Autodesk Fusion 360 part; units mm, degrees
(part 3 of 3)
  spline S38 degree 5 poles (8.1024, -6.5353) (8.1055, -6.5377) (8.1117, -6.5426) (8.1212, -6.5498) (8.1342, -6.5589) (8.1508, -6.5697) (8.1678, -6.5801) (8.1849, -6.5902) (8.2022, -6.6002) (8.2195, -6.6101) (8.237, -6.6198) (8.2545, -6.6295) (8.2721, -6.639) (8.2899, -6.6483) (8.3078, -6.6574) (8.3259, -6.6663) (8.3441, -6.6751) (8.3624, -6.6837) (8.3807, -6.6922) (8.3992, -6.7006) (8.4177, -6.7089) (8.4363, -6.717) (8.455, -6.725) (8.4738, -6.7329) (8.4927, -6.7407) (8.5116, -6.7484) (8.5307, -6.7559) (8.5498, -6.7633) (8.569, -6.7706) (8.5882, -6.7778) (8.6075, -6.7849) (8.6269, -6.7919) (8.6464, -6.7988) (8.6659, -6.8056) (8.6855, -6.8123) (8.7052, -6.8189) (8.7249, -6.8254) (8.7447, -6.8318) (8.7645, -6.838) (8.7845, -6.8442) (8.8044, -6.8503) (8.8245, -6.8563) (8.8446, -6.8622) (8.8647, -6.868) (8.8849, -6.8737) (8.9052, -6.8794) (8.9255, -6.8849) (8.9459, -6.8903) (8.9663, -6.8957) (8.9868, -6.9009) (9.0073, -6.9061) (9.0279, -6.9112) (9.0485, -6.9162) (9.0692, -6.9211) (9.0899, -6.9259) (9.1107, -6.9306) (9.1316, -6.9352) (9.1524, -6.9398) (9.1734, -6.9442) (9.1944, -6.9486) (9.2154, -6.9529) (9.2365, -6.9571) (9.2576, -6.9613) (9.2787, -6.9653) (9.3, -6.9693) (9.3212, -6.9731) (9.3425, -6.9769) (9.3638, -6.9806) (9.3852, -6.9842) (9.4067, -6.9878) (9.4281, -6.9912) (9.4453, -6.994) (9.4583, -6.9959) (9.4669, -6.9973) (9.4712, -6.9979) knots 0 0 0 0 0 0 0.01428571 0.02857143 0.04285714 0.05714286 0.07142857 0.08571429 0.1 0.11428571 0.12857143 0.14285714 0.15714286 0.17142857 0.18571429 0.2 0.21428571 0.22857143 0.24285714 0.25714286 0.27142857 0.28571429 0.3 0.31428571 0.32857143 0.34285714 0.35714286 0.37142857 0.38571429 0.4 0.41428571 0.42857143 0.44285714 0.45714286 0.47142857 0.48571429 0.5 0.51428571 0.52857143 0.54285714 0.55714286 0.57142857 0.58571429 0.6 0.61428571 0.62857143 0.64285714 0.65714286 0.67142857 0.68571429 0.7 0.71428571 0.72857143 0.74285714 0.75714286 0.77142857 0.78571429 0.8 0.81428571 0.82857143 0.84285714 0.85714286 0.87142857 0.88571429 0.9 0.91428571 0.92857143 0.94285714 0.95714286 0.97142857 0.98571429 1 1 1 1 1 1
  arc A78 (9.4712, -6.9979) -> (9.9744, -6.2599) centre (0, 0) ccw
  spline S39 degree 5 poles (9.9744, -6.2599) (9.9722, -6.2561) (9.9678, -6.2485) (9.9613, -6.2372) (9.9524, -6.2222) (9.9414, -6.2035) (9.9303, -6.1848) (9.9191, -6.1662) (9.9078, -6.1477) (9.8965, -6.1293) (9.8851, -6.1109) (9.8737, -6.0926) (9.8622, -6.0744) (9.8507, -6.0563) (9.8391, -6.0382) (9.8274, -6.0202) (9.8156, -6.0022) (9.8038, -5.9844) (9.792, -5.9666) (9.78, -5.9489) (9.768, -5.9313) (9.756, -5.9137) (9.7439, -5.8963) (9.7317, -5.8789) (9.7194, -5.8616) (9.7071, -5.8444) (9.6948, -5.8272) (9.6823, -5.8101) (9.6698, -5.7932) (9.6572, -5.7763) (9.6446, -5.7595) (9.6319, -5.7427) (9.6191, -5.7261) (9.6063, -5.7096) (9.5934, -5.6931) (9.5804, -5.6767) (9.5674, -5.6605) (9.5543, -5.6443) (9.5411, -5.6282) (9.5279, -5.6122) (9.5146, -5.5963) (9.5012, -5.5805) (9.4877, -5.5648) (9.4742, -5.5492) (9.4606, -5.5337) (9.4469, -5.5183) (9.4332, -5.503) (9.4194, -5.4878) (9.4055, -5.4728) (9.3915, -5.4578) (9.3775, -5.443) (9.3633, -5.4282) (9.3491, -5.4136) (9.3348, -5.3992) (9.3204, -5.3848) (9.306, -5.3706) (9.2914, -5.3565) (9.2768, -5.3425) (9.2621, -5.3286) (9.2473, -5.3149) (9.2324, -5.3013) (9.2174, -5.288) (9.2022, -5.2748) (9.1869, -5.2619) (9.1715, -5.2491) (9.1561, -5.2364) (9.1405, -5.2239) (9.1249, -5.2115) (9.1092, -5.1992) (9.0934, -5.1872) (9.0772, -5.1757) (9.064, -5.1669) (9.0539, -5.1607) (9.0471, -5.1567) (9.0436, -5.1547) knots -1 -1 -1 -1 -1 -1 -0.98571429 -0.97142857 -0.95714286 -0.94285714 -0.92857143 -0.91428571 -0.9 -0.88571429 -0.87142857 -0.85714286 -0.84285714 -0.82857143 -0.81428571 -0.8 -0.78571429 -0.77142857 -0.75714286 -0.74285714 -0.72857143 -0.71428571 -0.7 -0.68571429 -0.67142857 -0.65714286 -0.64285714 -0.62857143 -0.61428571 -0.6 -0.58571429 -0.57142857 -0.55714286 -0.54285714 -0.52857143 -0.51428571 -0.5 -0.48571429 -0.47142857 -0.45714286 -0.44285714 -0.42857143 -0.41428571 -0.4 -0.38571429 -0.37142857 -0.35714286 -0.34285714 -0.32857143 -0.31428571 -0.3 -0.28571429 -0.27142857 -0.25714286 -0.24285714 -0.22857143 -0.21428571 -0.2 -0.18571429 -0.17142857 -0.15714286 -0.14285714 -0.12857143 -0.11428571 -0.1 -0.08571429 -0.07142857 -0.05714286 -0.04285714 -0.02857143 -0.01428571 0 0 0 0 0 0
  line L39 (9.0436, -5.1547) -> (8.7512, -4.9877)
  arc A79 (8.5022, -4.176) -> (8.7512, -4.9877) centre (9.0587, -4.4493) ccw
  arc A80 (8.5022, -4.176) -> (8.566, -4.0436) centre (0, 0) ccw
  arc A81 (9.3558, -3.7322) -> (8.566, -4.0436) centre (9.1266, -4.3083) ccw
  line L40 (9.3558, -3.7322) -> (9.6687, -3.8567)
  spline S40 degree 5 poles (9.6687, -3.8567) (9.6724, -3.8582) (9.6798, -3.861) (9.691, -3.865) (9.7061, -3.8699) (9.7252, -3.8753) (9.7444, -3.8802) (9.7638, -3.8848) (9.7832, -3.8893) (9.8027, -3.8936) (9.8223, -3.8979) (9.8418, -3.9019) (9.8615, -3.9058) (9.8812, -3.9095) (9.9011, -3.9129) (9.921, -3.9161) (9.9409, -3.9191) (9.9609, -3.9219) (9.981, -3.9246) (10.0011, -3.9272) (10.0212, -3.9296) (10.0414, -3.9319) (10.0616, -3.9341) (10.0819, -3.9361) (10.1022, -3.938) (10.1226, -3.9397) (10.143, -3.9413) (10.1635, -3.9427) (10.1839, -3.9441) (10.2045, -3.9453) (10.225, -3.9464) (10.2456, -3.9474) (10.2662, -3.9482) (10.2869, -3.9489) (10.3076, -3.9496) (10.3283, -3.9501) (10.3491, -3.9504) (10.3699, -3.9507) (10.3907, -3.9509) (10.4116, -3.9509) (10.4324, -3.9508) (10.4534, -3.9507) (10.4743, -3.9504) (10.4953, -3.95) (10.5162, -3.9495) (10.5373, -3.9489) (10.5583, -3.9482) (10.5794, -3.9474) (10.6005, -3.9465) (10.6216, -3.9454) (10.6427, -3.9443) (10.6639, -3.9431) (10.6851, -3.9418) (10.7063, -3.9404) (10.7275, -3.9389) (10.7488, -3.9373) (10.7701, -3.9355) (10.7914, -3.9337) (10.8127, -3.9318) (10.834, -3.9298) (10.8554, -3.9277) (10.8768, -3.9256) (10.8982, -3.9233) (10.9196, -3.9209) (10.941, -3.9184) (10.9625, -3.9159) (10.9839, -3.9132) (11.0054, -3.9105) (11.0269, -3.9076) (11.0484, -3.9047) (11.07, -3.9017) (11.0872, -3.8992) (11.1001, -3.8973) (11.1088, -3.896) (11.1131, -3.8953) knots 0 0 0 0 0 0 0.01428571 0.02857143 0.04285714 0.05714286 0.07142857 0.08571429 0.1 0.11428571 0.12857143 0.14285714 0.15714286 0.17142857 0.18571429 0.2 0.21428571 0.22857143 0.24285714 0.25714286 0.27142857 0.28571429 0.3 0.31428571 0.32857143 0.34285714 0.35714286 0.37142857 0.38571429 0.4 0.41428571 0.42857143 0.44285714 0.45714286 0.47142857 0.48571429 0.5 0.51428571 0.52857143 0.54285714 0.55714286 0.57142857 0.58571429 0.6 0.61428571 0.62857143 0.64285714 0.65714286 0.67142857 0.68571429 0.7 0.71428571 0.72857143 0.74285714 0.75714286 0.77142857 0.78571429 0.8 0.81428571 0.82857143 0.84285714 0.85714286 0.87142857 0.88571429 0.9 0.91428571 0.92857143 0.94285714 0.95714286 0.97142857 0.98571429 1 1 1 1 1 1
  arc A82 (11.1131, -3.8953) -> (11.3764, -3.0418) centre (0, 0) ccw
  spline S41 degree 5 poles (11.3764, -3.0418) (11.3732, -3.0388) (11.3668, -3.0329) (11.3572, -3.024) (11.3443, -3.0122) (11.3282, -2.9976) (11.3121, -2.9831) (11.2959, -2.9686) (11.2797, -2.9542) (11.2635, -2.9399) (11.2472, -2.9257) (11.2309, -2.9116) (11.2145, -2.8976) (11.1981, -2.8837) (11.1817, -2.8698) (11.1652, -2.856) (11.1487, -2.8424) (11.1322, -2.8288) (11.1156, -2.8153) (11.099, -2.8019) (11.0823, -2.7886) (11.0657, -2.7754) (11.0489, -2.7623) (11.0322, -2.7492) (11.0154, -2.7363) (10.9985, -2.7235) (10.9816, -2.7107) (10.9647, -2.6981) (10.9478, -2.6856) (10.9308, -2.6731) (10.9138, -2.6608) (10.8967, -2.6486) (10.8796, -2.6364) (10.8624, -2.6244) (10.8453, -2.6125) (10.8281, -2.6007) (10.8108, -2.5889) (10.7935, -2.5773) (10.7762, -2.5659) (10.7588, -2.5545) (10.7414, -2.5432) (10.724, -2.532) (10.7065, -2.521) (10.689, -2.5101) (10.6714, -2.4993) (10.6538, -2.4886) (10.6362, -2.4781) (10.6185, -2.4676) (10.6008, -2.4573) (10.583, -2.4471) (10.5652, -2.4371) (10.5474, -2.4272) (10.5295, -2.4174) (10.5115, -2.4078) (10.4936, -2.3983) (10.4755, -2.389) (10.4575, -2.3798) (10.4394, -2.3707) (10.4213, -2.3618) (10.4031, -2.3531) (10.3848, -2.3445) (10.3665, -2.3361) (10.3482, -2.328) (10.3298, -2.3202) (10.3113, -2.3125) (10.2928, -2.305) (10.2742, -2.2976) (10.2556, -2.2903) (10.237, -2.2832) (10.2183, -2.2765) (10.1995, -2.2702) (10.1843, -2.2657) (10.1728, -2.2627) (10.1651, -2.2609) (10.1612, -2.26) knots -1 -1 -1 -1 -1 -1 -0.98571429 -0.97142857 -0.95714286 -0.94285714 -0.92857143 -0.91428571 -0.9 -0.88571429 -0.87142857 -0.85714286 -0.84285714 -0.82857143 -0.81428571 -0.8 -0.78571429 -0.77142857 -0.75714286 -0.74285714 -0.72857143 -0.71428571 -0.7 -0.68571429 -0.67142857 -0.65714286 -0.64285714 -0.62857143 -0.61428571 -0.6 -0.58571429 -0.57142857 -0.55714286 -0.54285714 -0.52857143 -0.51428571 -0.5 -0.48571429 -0.47142857 -0.45714286 -0.44285714 -0.42857143 -0.41428571 -0.4 -0.38571429 -0.37142857 -0.35714286 -0.34285714 -0.32857143 -0.31428571 -0.3 -0.28571429 -0.27142857 -0.25714286 -0.24285714 -0.22857143 -0.21428571 -0.2 -0.18571429 -0.17142857 -0.15714286 -0.14285714 -0.12857143 -0.11428571 -0.1 -0.08571429 -0.07142857 -0.05714286 -0.04285714 -0.02857143 -0.01428571 0 0 0 0 0 0
  line L41 (10.1612, -2.26) -> (9.8326, -2.1866)
  arc A83 (9.3554, -1.4844) -> (9.8326, -2.1866) centre (9.9677, -1.5815) ccw
  circle A84 centre (0, 0) radius 3.625
  circle A85 centre (0, 0) radius 3.625
  circle A86 centre (0, 0) radius 4.875
  dimension "d12" = 1.25
  constraint concentric A0 A85
extrude "Extrude4" add sketch "Sketch2 (2)" along normal blind 7 contours A86 in component "Spur Gear (21 teeth)"
extrude "Extrude5" add sketch "Sketch1 (2)" along normal blind 14 contours A0 L0 L1 picked at (-3.0023, 0) in component "Spur Gear (21 teeth)"
extrude "Extrude6" cut 1 faces at (2.8986, -7.3856, 7) along direction (0, 0, -1) blind 1 in component "Spur Gear (21 teeth)"
extrude "Extrude7" cut 1 faces at (-2.8083, 0, 14) along direction (0, 0, -1) blind 1 in component "Spur Gear (21 teeth)"
component "Spur Gear (21 teeth)" placed x (1, 0, 0) y (0, 1, 0) z (0, 0, 1) at (0, 0, 0)
